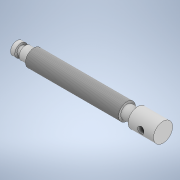
# Autodesk Inventor part: haste_roscada
Saved by Autodesk Inventor 2020 (Build 240168000, 168)
## iProperties
Created: 2022-03-09
Part Number: haste_roscada
Material: Genérico
Document SubType Name: Modeling
Designer: 19710060
Density: 1 g/cm^3
Appearance: Padrão
Author: 19710060
Autodesk Inventor part; units mm, degrees
ref_plane "YZ Plane" through (0, 0, 0) normal (1, 0, 0) x (0, 1, 0)
ref_plane "XZ Plane" through (0, 0, 0) normal (0, 1, 0) x (-1, 0, 0)
ref_plane "XY Plane" through (0, 0, 0) normal (0, 0, 1) x (1, 0, 0)
sketch "Esboço1" plane through (0, 0, 0) normal (0, 0, 1) x (1, 0, 0)
  line L0 (0, 0) -> (0, 6)
  line L1 (0, 6) -> (4, 6)
  line L2 (4, 6) -> (4, 4)
  line L3 (4, 4) -> (8, 4)
  line L4 (8, 4) -> (8, 6)
  line L5 (8, 6) -> (16, 6)
  line L6 (16, 6) -> (16, 8)
  line L7 (16, 8) -> (104, 8)
  line L8 (104, 8) -> (104, 6)
  line L9 (104, 6) -> (114, 6)
  line L10 (114, 6) -> (114, 9)
  line L11 (114, 9) -> (138, 9)
  line L12 (138, 9) -> (138, 0)
  line L13 (138, 0) -> (0, 0)
  dimension "d0" = 6
  dimension "d1" = 4
  dimension "d2" = 2
  dimension "d3" = 4
  dimension "d4" = 2
  dimension "d5" = 8
  dimension "d6" = 2
  dimension "d7" = 88
  dimension "d11" = 2
  dimension "d12" = 10
  dimension "d13" = 3
  dimension "d14" = 24
  constraints: 28 end point, 9 perpendicular, 2 point on line, 2 vertical, 1 horizontal
  measures "d0" distance of L0.start L0.end
  measures "d1" distance of L0.end L1.end
  measures "d2" distance of L1.end L2.end
  measures "d3" distance of L2.end L3.end
  measures "d4" distance of L3.end L4.end
  measures "d5" distance of L4.end L5.end
  measures "d6" distance of L5.end L6.end
  measures "d7" distance of L6.end L7.end
  measures "d11" distance of L7.end L8.end
  measures "d12" distance of L8.end L9.end
  measures "d13" distance of L9.end L10.end
  measures "d14" distance of L10.end L11.end
revolve "Revolução1" add sketch "Esboço1" angle 360 about axis through (138, 0, 0) along (-1, 0, 0)
sketch "Esboço2" plane through (0, 0, 0) normal (0, 0, 1) x (1, 0, 0)
  line L0 (138, -9) -> (138, 9) projected
  line L1 (138, 0) -> (126, 0)
  point P0 (0, 0)
  dimension "d16" = 12
  constraints: 2 end point, 1 coincident, 1 horizontal, 1 midpoint
  measures "d16" distance of L1.start L1.end
hole "Furo1" at (126, 0, 0) direction (0, 0, -1) diameter 6 end through all both
thread "Rosca1" size "M16x1" class "6g" standard "ANSI Metric M Profile" full length
